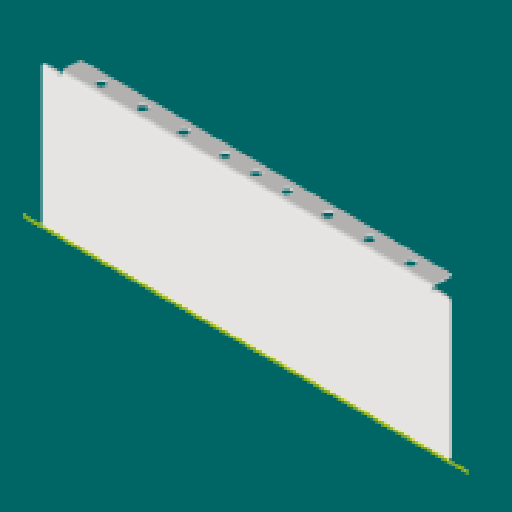
# Autodesk Inventor part: P_TYŁ
Saved by Autodesk Inventor 2023 (Build 270158000, 158)
## iProperties
Created: 2023-01-28
Part Number: P_TYŁ
Material: Generic
Document SubType Name: Sheet Metal
Designer: HeavyDrewno
Density: 1 g/cm^3
Sheet Metal Rule: Default
Appearance: Default
Author: HeavyDrewno
Autodesk Inventor part; units mm, degrees
ref_plane "YZ Plane" through (0, 0, 0) normal (1, 0, 0) x (0, 1, 0)
ref_plane "XZ Plane" through (0, 0, 0) normal (0, 1, 0) x (-1, 0, 0)
ref_plane "XY Plane" through (0, 0, 0) normal (0, 0, 1) x (1, 0, 0)
ref_plane "Work Plane1" through (0, 0, 0) normal (0, 0, 1) x (1, 0, 0)
sketch "Sketch1" plane through (0, 0, 0) normal (0, 0, 1) x (1, 0, 0)
  line L0 (-398, 4) -> (-398, 136)
  arc A0 (-398, 4) -> (-396, 2) centre (-396, 4) ccw
  line L1 (-4, 2) -> (-396, 2)
  arc A1 (-4, 2) -> (-2, 4) centre (-4, 4) ccw
  line L2 (-2, 4) -> (-2, 136)
  arc A2 (-2, 136) -> (-4, 138) centre (-4, 136) ccw
  line L3 (-20, 138) -> (-4, 138)
  arc A3 (-396, 138) -> (-398, 136) centre (-396, 136) ccw
  line L4 (-380, 138) -> (-396, 138)
  line L5 (-20, 138) -> (-380, 138)
  point P0 (0, 0)
extrude "Plate1" add sketch "Sketch1" against normal blind 2
sketch "Sketch2" plane through (-396, 138, 0) normal (0, 1, 0) x (1, 0, 0)
  line L0 (376, 0) -> (376, 1000) construction
  line L1 (16, 0) -> (16, 1000) construction
  line L2 (396, 1000) -> (396, 0)
  line L3 (16, 0) -> (16, 20)
  line L4 (16, 20) -> (376, 20)
  line L5 (376, 0) -> (376, 20)
  line L6 (376, 0) -> (16, 0)
  line L7 (392, 0) -> (0, 0)
  dimension "d2" = 20
  measures "d2" distance of L1.start L3.end
sheet face with bend "Face2" sketch "Sketch2" thickness 2 toward (0, 1, 0) bend radius 2 relief straight relief width 2 relief depth 1
bend "Bend1"
sketch "Sketch3" plane through (-396, 140, 0) normal (0, 1, 0) x (1, 0, 0)
  line L0 (376, 0) -> (16, 0) projected
  circle A0 centre (6, 10) radius 4.5 construction
  circle A1 centre (386, 10) radius 4.5 construction
  point P0 (396, 0)
  point P1 (46, 10)
  point P2 (86, 10)
  point P3 (126, 10)
  point P4 (166, 10)
  point P5 (196, 10)
  point P6 (226, 10)
  point P7 (266, 10)
  point P8 (306, 10)
  point P9 (346, 10)
  dimension "d8" = 10
  dimension "d9" = 40
  dimension "d10" = 40
  dimension "d11" = 40
  dimension "d12" = 40
  dimension "d13" = 30
  dimension "d14" = 40
  dimension "d15" = 40
  dimension "d16" = 40
  dimension "d17" = 40
  measures "d8" distance from line of L0 point (46, 10)
  measures "d9" distance of A0.centre point (46, 10)
  measures "d10" distance of point (46, 10) point (86, 10)
  measures "d11" distance of point (126, 10) point (86, 10)
  measures "d12" distance of point (166, 10) point (126, 10)
  measures "d13" distance of point (166, 10) point (196, 10)
  measures "d14" distance of point (346, 10) A1.centre
  measures "d15" distance of point (306, 10) point (346, 10)
  measures "d16" distance of point (266, 10) point (306, 10)
  measures "d17" distance of point (226, 10) point (266, 10)
hole "Hole1" at (-350, 140, -10) at (-310, 140, -10) at (-270, 140, -10) at (-230, 140, -10) at (-200, 140, -10) at (-170, 140, -10) at (-130, 140, -10) at (-90, 140, -10) at (-50, 140, -10) direction (0, -1, 0) diameter 9 depth 2 tip angle 118
equation "\"d23\" = Thickness"
equation "\"d0\" = Thickness"
equation "\"d3\" = BendRadius"
equation "\"d4\" = BendReliefWidth"
equation "\"d6\" = MinimumRemnant"
equation "\"d5\" = BendReliefDepth"
equation "\"d7\" = TransitionRadius"
equation "\"BendRadius\" = Thickness"
equation "\"BendReliefWidth\" = Thickness"
equation "\"BendReliefDepth\" = 0.5 * Thickness"
equation "\"CornerReliefSize\" = 4 * Thickness"
equation "\"MinimumRemnant\" = 2 * Thickness"
equation "\"TransitionRadius\" = BendRadius"
equation "\"JacobiRadiusSize\" = BendRadius"
equation "\"GapSize\" = Thickness"
equation "\"Thickness\" = 2"
body "Solid1"
